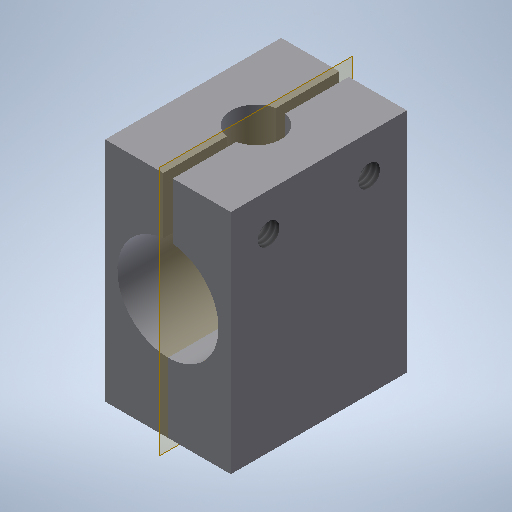
# Autodesk Inventor part: Galvo-Holder-PolarisMount_metal_v2
Saved by Autodesk Inventor 2025.2 (Build 292293000, 293)
## iProperties
Created: 2014-07-28
Part Number: Galvo-Holder-PolarisMount_metal_v2
Material: Generic
Document SubType Name: Modeling
Designer: 120pa
Density: 1 g/cm^3
Appearance: Default
Mass: 11.544 g
Surface Area: 64.1947 cm^2
Volume: 11.544 cm^3
Author: 120pa
Autodesk Inventor part; units mm, degrees
ref_plane "YZ Plane" through (0, 0, 0) normal (1, 0, 0) x (0, 1, 0)
ref_plane "XZ Plane" through (0, 0, 0) normal (0, 1, 0) x (-1, 0, 0)
ref_plane "XY Plane" through (0, 0, 0) normal (0, 0, 1) x (1, 0, 0)
sketch "Sketch1" plane through (0, 0, 0) normal (0, 1, 0) x (-1, 0, 0)
  line L0 (-12.788, 8.8746) -> (7.212, 8.8746)
  line L1 (7.212, 8.8746) -> (7.212, -27.2254)
  line L2 (7.212, -27.2254) -> (-12.788, -27.2254)
  line L3 (-12.788, -27.2254) -> (-12.788, 8.8746)
  point P0 (0, 0)
  dimension "d0" = 20
  dimension "d1" = 36.1
  constraints: 8 end point, 3 perpendicular
  measures "d0" distance of L0.start L0.end
  measures "d1" distance of L0.end L1.end
extrude "Extrusion1" add sketch "Sketch1" along normal blind 28
sketch "Sketch2" plane through (0, 0, 0) normal (0, -1, 0) x (1, 0, 0)
  line L0 (-7.212, -27.2254) -> (12.788, -27.2254) projected
  line L1 (12.788, -27.2254) -> (12.788, 8.8746) projected
  circle A0 centre (2.788, -8.1254) radius 8.05
  point P0 (0, 0)
  dimension "d4" = 10
  dimension "d5" = 16.1
  dimension "d6" = 19.1
  constraints: 1 centre point
  measures "d4" distance from line of L1 A0.centre
  measures "d5" diameter of A0
  measures "d6" distance from line of A0.centre L0
extrude "Extrusion2" cut sketch "Sketch2" against normal blind 30
sketch "Sketch3" plane through (0, 0, 0) normal (0, -1, 0) x (1, 0, 0)
  circle A0 centre (2.788, -8.1254) radius 8.05 projected
  line L0 (12.788, 8.8746) -> (-7.212, 8.8746) projected
  line L1 (2.038, 8.8746) -> (3.538, 8.8746)
  line L2 (3.538, 8.8746) -> (3.538, -9.1254)
  line L3 (3.538, -9.1254) -> (2.038, -9.1254)
  line L4 (2.038, -9.1254) -> (2.038, 8.8746)
  point P0 (0, 0)
  dimension "d9" = 18
  dimension "d11" = 1.5
  dimension "d12" = 0.75
  constraints: 8 end point, 1 point on line
  measures "d9" distance of L1.end L2.end
  measures "d11" distance between parallel lines of L2 L4
  measures "d12" distance from line of L2 A0.centre
extrude "Extrusion3" cut sketch "Sketch3" against normal blind 30 contours L2 L3 L4 A0 | A0 L4 L0 L2 picked at (2.8714, -6.11)
sketch "Sketch4" plane through (12.788, 0, -27.2254) normal (0, 0, -1) x (-1, 0, 0)
  line L0 (0, 28) -> (20, 28) projected
  line L1 (0, 0) -> (0, 28) projected
  circle A0 centre (10, 14) radius 2.286
  point P0 (12.788, 0)
  dimension "d15" = 14
  dimension "d16" = 10
  dimension "d17" = 4.572
  constraints: 1 centre point
  measures "d15" distance from line of L0 A0.centre
  measures "d16" distance from line of L1 A0.centre
  measures "d17" diameter of A0
extrude "Extrusion4" cut sketch "Sketch4" against normal blind 10
sketch "Sketch6" plane through (-7.212, 0, -27.2254) normal (-1, 0, 0) x (0, 0, 1)
  line L0 (36.1, 0) -> (0, 0) projected
  line L1 (36.1, 0) -> (36.1, 28) projected
  line L2 (0, 28) -> (36.1, 28) projected
  circle A0 centre (30.1, 6) radius 2.49
  circle A1 centre (30.1, 22) radius 2.49
  point P0 (27.2254, 0)
  dimension "d20" = 6
  dimension "d21" = 6
  dimension "d22" = 4.98
  dimension "d23" = 4.98
  dimension "d24" = 6
  dimension "d25" = 6
  constraints: 2 centre point
  measures "d20" distance from line of L1 A1.centre
  measures "d21" distance from line of L1 A0.centre
  measures "d22" diameter of A1
  measures "d23" diameter of A0
  measures "d24" distance from line of A1.centre L2
  measures "d25" distance from line of A0.centre L0
extrude "Extrusion5" cut sketch "Sketch6" against normal blind 10
sketch "Sketch7" plane through (12.788, 0, 8.8746) normal (1, 0, 0) x (0, 0, -1)
  circle A0 centre (6, 6) radius 1.725
  circle A1 centre (6, 22) radius 1.725
  line L0 (36.1, 0) -> (0, 0) projected
  line L1 (0, 28) -> (36.1, 28) projected
  line L2 (0, 0) -> (0, 28) projected
  point P0 (8.8746, 0)
  dimension "d28" = 3.45
  dimension "d29" = 3.45
  dimension "d88" = 6
  dimension "d89" = 6
  dimension "d91" = 6
  dimension "d92" = 6
  constraints: 2 centre point, 2 coincident
  measures "d28" diameter of A0
  measures "d29" diameter of A1
  measures "d88" distance from line of L0 A0.centre
  measures "d89" distance from line of L1 A1.centre
  measures "d91" distance from line of L2 A0.centre
  measures "d92" distance from line of L2 A1.centre
extrude "Extrusion8" cut sketch "Sketch7" against normal blind 10
thread "Thread8" size "8-32 UNC" class "2B" standard "ANSI Unified Screw Threads" full length
thread "Thread11" size "8-32 UNC" class "2B" standard "ANSI Unified Screw Threads" full length
sketch "Sketch11" plane through (12.788, 0, -27.2254) normal (0, 0, -1) x (-1, 0, 0)
  circle A0 centre (10, 14) radius 2.286 projected
  circle A1 centre (10, 14) radius 0.7841
  circle A2 centre (10, 9) radius 1.0109
  line L0 (10, 18) -> (10, 17) construction
  line L1 (11.0033, 17) -> (11.0033, 18)
  point P0 (12.788, 0)
  point P1 (10, 17.5)
  dimension "d69" = 5
  dimension "d71" = 2.0218
  constraints: 6 end point, 2 centre point, 2 coincident, 1 midpoint, 1 vertical
  measures "d69" distance of A1.centre point (10, 9)
  measures "d71" diameter of A2
hole "Hole1" at (2.788, 9, -27.2254) direction (0, 0, 1) diameter 2.0218 depth 1.91 tip angle 118
sketch "Sketch13" plane through (12.788, 0, -27.2254) normal (0, 0, -1) x (-1, 0, 0)
  circle A0 centre (10, 9) radius 1.0109 projected
  line L0 (10, 18.5) -> (10, 19.5) construction
  line L1 (11.0109, 18.5) -> (11.0109, 19.5)
  line L2 (8.9891, 19.5) -> (8.9891, 18.5)
  arc A1 (8.9891, 18.5) -> (11.0109, 18.5) centre (10, 18.5) ccw
  arc A2 (11.0109, 19.5) -> (8.9891, 19.5) centre (10, 19.5) ccw
  point P0 (12.788, 0)
  point P1 (10, 19)
  dimension "d81" = 0.5
  dimension "d82" = 2.0218
  dimension "d97" = 10
  constraints: 8 end point, 4 point on circle, 4 tangent, 2 centre point, 1 coincident, 1 midpoint, 1 parallel, 1 vertical
  measures "d81" distance of point (10, 19) L0.end
  measures "d82" diameter of A2
  measures "d97" distance of A0.centre point (10, 19)
extrude "Extrusion12" cut sketch "Sketch13" against normal blind 1.91 contours A1 L2 A2 L1
sketch "Sketch15" plane through (-7.212, 0, -27.2254) normal (-1, 0, 0) x (0, 0, 1)
  circle A0 centre (30.1, 22) radius 1.725 projected
  circle A1 centre (30.1, 22) radius 3.9688
  circle A2 centre (30.1, 6) radius 1.725 projected
  circle A3 centre (30.1, 6) radius 3.9687
  point P0 (27.2254, 0)
  point P1 (27.015, 20.5839)
  point P2 (27.015, 23.4161)
  point P3 (27.015, 4.5839)
  point P4 (27.015, 7.4161)
  dimension "d93" = 7.9375
  dimension "d94" = 7.9375
  constraints: 2 centre point, 2 coincident, 2 other
  measures "d93" diameter of A1
  measures "d94" diameter of A3
extrude "Extrusion13" cut sketch "Sketch15" against normal blind 4.572 contours A0 | A1 | A2 | A3
sketch "Sketch16" plane through (-7.212, 0, 8.8746) normal (0, 0, 1) x (1, 0, 0)
  circle A0 centre (10, 14) radius 2.286 projected
  circle A1 centre (10, 14) radius 3.9687
  point P0 (7.212, 0)
  dimension "d98" = 7.9375
  constraints: 1 centre point, 1 coincident
  measures "d98" diameter of A1
extrude "Extrusion14" cut sketch "Sketch16" against normal blind 29.622 contours A0 | A1
ref_plane "Work Plane1" through (2.788, 28, 8.8746) normal (1, 0, 0) x (0, 0, -1)
body "Solid1"
